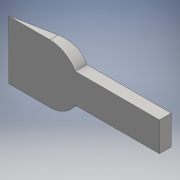
# Autodesk Inventor part: Scooper-1
Saved by Autodesk Inventor 2016 (Build 200138000, 138)
## iProperties
Created: 2017-07-07
Part Number: Scooper-1
Material: Generic
Document SubType Name: Modeling
Designer: alex
Density: 1 g/cm^3
Appearance: Default
Author: alex
Autodesk Inventor part; units mm, degrees
ref_plane "YZ Plane" through (0, 0, 0) normal (1, 0, 0) x (0, 1, 0)
ref_plane "XZ Plane" through (0, 0, 0) normal (0, 1, 0) x (-1, 0, 0)
ref_plane "XY Plane" through (0, 0, 0) normal (0, 0, 1) x (1, 0, 0)
sketch "Sketch1" plane through (0, 0, 0) normal (0, 1, 0) x (-1, 0, 0)
  line L0 (7, 5) -> (0, 5)
  line L1 (0, -5) -> (7, -5)
  line L2 (7, -5) -> (7, 5)
  arc A0 (0, 5) -> (0, -5) centre (0, 0) ccw
  dimension "d0" = 10
  dimension "d2" = 7
  constraints: 6 end point, 3 coincident, 2 point on circle, 2 tangent, 1 centre point, 1 horizontal, 1 parallel, 1 vertical
  measures "d0" distance between parallel lines of L1 L0
  measures "d2" distance from line of point (0, 0) L2
extrude "Extrusion1" add sketch "Sketch1" along normal blind 2
chamfer "Chamfer1" distance 10 angle 11 1 edges at (-7, 2, 0) measured on face at (-6.5, 2, 0)
ref_plane "Work Plane1" through (3, 2, 4) normal (0, 1, 0) x (1, 0, 0)
sketch "Sketch3" plane through (3, 2, 4) normal (0, 1, 0) x (1, 0, 0)
  arc A0 (-2.356, 0.3478) -> (-2.8364, 7.7049) centre (-3, 4) ccw
  line L0 (-10, -1) -> (-3, -1) projected
  line L1 (-2.356, 0.3478) -> (-10, -1)
  line L2 (-3, 9) -> (-10, 9) projected
  line L3 (-10, 9) -> (-2.356, 7.6522)
  line L4 (-10, 9) -> (-10, -1)
  dimension "d18" = 10
  constraints: 6 end point, 3 point on circle, 2 tangent, 1 centre point, 1 coincident, 1 vertical
  measures "d18" angle of L2 L3
extrude "Extrusion2" cut sketch "Sketch3" against normal blind 1.1
chamfer "Chamfer2" distance 3 angle 45 1 edges at (-2.659, 0.9, 0)
sketch "Sketch4" plane through (0, 0, 0) normal (0, 1, 0) x (-1, 0, 0)
  line L0 (-3.7085, -2.5) -> (-18.7085, -2.5)
  line L1 (-18.7085, -2.5) -> (-18.7085, 2.5)
  line L2 (-18.7085, 2.5) -> (-3.7085, 2.5)
  line L3 (-3.7085, 2.5) -> (-3.7085, -2.5)
  arc A0 (-3, 2.1801) -> (-3, -2.1801) centre (0, 0) ccw projected
  arc A1 (-3, 4) -> (-3, -4) centre (0, 0) ccw projected
  point P0 (-3.7085, 0)
  point P1 (-3.7085, 0)
  point P2 (-18.7085, 0)
  point P3 (-5, 0)
  dimension "d24" = 5
  dimension "d25" = 15
  constraints: 8 end point, 2 midpoint, 2 parallel, 2 point on circle, 1 coincident, 1 horizontal, 1 horizontal alignment, 1 perpendicular
  measures "d24" distance between parallel lines of L2 L0
  measures "d25" distance of L0.start L0.end
extrude "Extrusion3" add sketch "Sketch4" along normal blind 2
body "Solid1"
